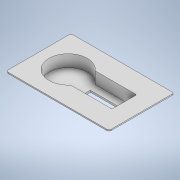
# Autodesk Inventor part: badge
Saved by Autodesk Inventor 2022 (Build 260153000, 153)
## iProperties
Created: 2019-12-22
Part Number: badge
Material: Generic
Document SubType Name: Modeling
Designer: user
Density: 1 g/cm^3
Appearance: Default
Author: user
## iProperties of the stored document _3DPrint.ipt
Created: 2019-12-23
Part Number: _3DPrint
Material: Generic
Document SubType Name: Modeling
Designer: user
Density: 1 g/cm^3
Appearance: Default
Author: user
Autodesk Inventor part; units mm, degrees
ref_plane "YZ Plane" through (0, 0, 0) normal (1, 0, 0) x (0, 1, 0)
ref_plane "XZ Plane" through (0, 0, 0) normal (0, 1, 0) x (-1, 0, 0)
ref_plane "XY Plane" through (0, 0, 0) normal (0, 0, 1) x (1, 0, 0)
sketch "Sketch1" plane through (0, 0, 0) normal (0, 1, 0) x (-1, 0, 0)
  circle A0 centre (-14.0224, -4.7987) radius 17
  line L0 (-61.8084, 4.4628) -> (-61.8084, -14.0372)
  line L1 (-59.8084, -16.0372) -> (-26.7776, -16.0372)
  line L2 (-26.7573, 6.4628) -> (-59.8084, 6.4628)
  arc A1 (-61.8084, -14.0372) -> (-59.8084, -16.0372) centre (-59.8084, -14.0372) ccw
  arc A2 (-59.8084, 6.4628) -> (-61.8084, 4.4628) centre (-59.8084, 4.4628) ccw
  line L3 (-28.2727, -0.5372) -> (-54.8084, -0.5372)
  line L4 (-54.8084, -0.5372) -> (-54.8084, -9.0372)
  line L5 (-54.8084, -9.0372) -> (-28.2727, -9.0372)
  line L6 (-28.2727, -9.0372) -> (-28.2727, -0.5372)
  line L7 (8.6213, 22.2028) -> (-72.9787, 22.2028)
  line L8 (-73.8987, -31.7772) -> (8.6213, -31.7772)
  line L9 (10.6213, -29.7772) -> (10.6213, 20.2028)
  line L10 (-74.9787, 20.2028) -> (-74.9787, 4.3773)
  line L11 (-74.9787, -30.6972) -> (-74.9787, -14.8717)
  arc A3 (-74.9787, -30.6972) -> (-73.8987, -31.7772) centre (-73.8987, -30.6972) ccw
  arc A4 (-72.9787, 22.2028) -> (-74.9787, 20.2028) centre (-72.9787, 20.2028) ccw
  arc A5 (10.6213, 20.2028) -> (8.6213, 22.2028) centre (8.6213, 20.2028) ccw
  arc A6 (8.6213, -31.7772) -> (10.6213, -29.7772) centre (8.6213, -29.7772) ccw
  line L12 (-74.9787, 4.3773) -> (-74.9787, -14.8717)
  circle A7 centre (-14.0224, -4.7987) radius 16
  line L13 (-27.4955, -15.0372) -> (-59.8084, -15.0372)
  line L14 (-60.8084, -14.0372) -> (-60.8084, 4.4628)
  arc A8 (-60.8084, -14.0372) -> (-59.8084, -15.0372) centre (-59.8084, -14.0372) ccw
  line L15 (-59.8084, 5.4628) -> (-27.576, 5.4628)
  arc A9 (-59.8084, 5.4628) -> (-60.8084, 4.4628) centre (-59.8084, 4.4628) ccw
  line L16 (-26.7776, -16.0372) -> (-25.4108, -16.0372)
  line L17 (-27.4955, -15.0372) -> (-26.3176, -15.0372)
  line L18 (-27.576, 5.4628) -> (-26.2984, 5.4628)
  line L19 (-26.7573, 6.4628) -> (-25.388, 6.4628)
  point P0 (0, 0)
  point P1 (-61.8084, -16.0372)
  dimension "d20" = 34
  dimension "d26" = 2
  dimension "d28" = 7
  dimension "d32" = 7
  dimension "d167" = 8.5
  dimension "d171" = 26.5357
  dimension "d177" = 85.6
  dimension "d229" = 32
  dimension "d230" = 1
  dimension "d231" = 1
  dimension "d232" = 1
  dimension "d233" = 1
  dimension "d234" = 1
  dimension "d235" = 1
  dimension "d241" = 53.98
  dimension "d242" = 22.74
  dimension "d243" = 22.74
  dimension "d248" = 62.786
  dimension "d249" = 6
  constraints: 40 end point, 23 point on circle, 16 tangent, 10 centre point, 6 horizontal, 6 parallel, 3 perpendicular, 3 point on line, 3 vertical, 2 equal radius
  measures "d20" diameter of A0
  measures "d26" radius of A1
  measures "d28" distance between parallel lines of L1 L5
  measures "d32" distance between parallel lines of L3 L2
  measures "d167" distance between parallel lines of L3 L5
  measures "d171" distance between parallel lines of L4 L6
  measures "d177" distance between parallel lines of L11 L9
  measures "d229" diameter of A7
  measures "d230" radial gap between concentric circles of A0 A7
  measures "d231" distance between parallel lines of L13 L1
  measures "d232" distance between parallel lines of L0 L14
  measures "d233" radius of A8
  measures "d234" distance between parallel lines of L2 L15
  measures "d235" radius of A9
  measures "d241" distance between parallel lines of L8 L7
  measures "d242" distance between parallel lines of L8 L5
  measures "d243" distance between parallel lines of L7 L3
  measures "d249" distance between parallel lines of L4 L14
extrude "Extrusion22" add sketch "Sketch1" along normal blind 1
extrude "Extrusion23" add sketch "Sketch1" against normal blind 10.5 contours A0 L16 A7 L19 | L19 A7 L18 A0 | A0 L15 A9 L14 A8 L13 L1 A1 L0 A2 L2 | A0 L13 L17 A7 L16 | L18 A7 L3 A0 | A0 L3 L4 L5 L13 A8 L14 A9 L15 | A7 L5 L6 L3 | A0 L5 A7 L17 L13 picked at (-18.1893, -4.791)
extrude "Extrusion24" cut sketch "Sketch1" against normal blind 9 contours L18 A7 L3 A0 | A0 L3 L4 L5 L13 A8 L14 A9 L15 | A7 L5 L6 L3 | A0 L5 A7 L17 L13 picked at (-18.1893, -4.791)
extrude "Extrusion25" add sketch "Sketch1" along normal blind 1 contours A0 L16 A7 L19 | L19 A7 L18 A0 | A0 L15 A9 L14 A8 L13 L1 A1 L0 A2 L2 | A0 L13 L17 A7 L16
sketch "Sketch25" plane through (0, 0, 0) normal (0, -1, 0) x (1, 0, 0)
  line L0 (61.0662, 20.9281) -> (73.8693, 20.9281) construction
  line L1 (73.8693, 20.9281) -> (73.8693, 15.5184) construction
  line L2 (73.8693, 15.5184) -> (61.0662, 15.5184) construction
  line L3 (61.0662, 15.5184) -> (61.0662, 20.9281) construction
  line L4 (63.224, 20.0701) -> (62.3275, 17.6914)
  line L5 (62.3275, 17.6914) -> (61.9679, 17.6914)
  line L6 (61.9679, 17.6914) -> (61.079, 20.0701)
  line L7 (61.079, 20.0701) -> (61.5132, 20.0701)
  line L8 (61.5132, 20.0701) -> (62.1631, 18.2385)
  line L9 (62.1631, 18.2385) -> (62.8079, 20.0701)
  line L10 (62.8079, 20.0701) -> (63.224, 20.0701)
  line L11 (65.2637, 17.6914) -> (63.7173, 17.6914)
  line L12 (63.7173, 17.6914) -> (63.7173, 18.015)
  line L13 (63.7173, 18.015) -> (64.2927, 18.015)
  line L14 (64.2927, 18.015) -> (64.2927, 20.1395)
  line L15 (64.2927, 20.1395) -> (63.7173, 20.1395)
  line L16 (63.7173, 20.1395) -> (63.7173, 20.4298)
  spline S0 degree 2 poles (63.7173, 20.4298) (64.0435, 20.4298) (64.3518, 20.6147) (64.3723, 20.8716) knots 0 0 0 1 2 2 2
  line L17 (64.3723, 20.8716) -> (64.7011, 20.8716)
  line L18 (64.7011, 20.8716) -> (64.7011, 18.015)
  line L19 (64.7011, 18.015) -> (65.2637, 18.015)
  line L20 (65.2637, 18.015) -> (65.2637, 17.6914)
  line L21 (66.5276, 17.6914) -> (66.019, 17.6914)
  line L22 (66.019, 17.6914) -> (66.019, 18.2976)
  line L23 (66.019, 18.2976) -> (66.5276, 18.2976)
  line L24 (66.5276, 18.2976) -> (66.5276, 17.6914)
  spline S1 degree 2 poles (69.1402, 19.2764) (69.1402, 18.4235) (68.6444, 17.6246) (68.128, 17.6246) knots 0 0 0 1 2 2 2
  spline S2 degree 2 poles (68.128, 17.6246) (67.604, 17.6246) (67.1133, 18.4389) (67.1133, 19.2738) knots 0 0 0 1 2 2 2
  spline S3 degree 2 poles (67.1133, 19.2738) (67.1133, 20.1318) (67.6091, 20.9256) (68.128, 20.9256) knots 0 0 0 1 2 2 2
  spline S4 degree 2 poles (68.128, 20.9256) (68.6495, 20.9256) (69.1402, 20.1035) (69.1402, 19.2764) knots 0 0 0 1 2 2 2
  spline S5 degree 2 poles (68.5956, 18.3105) (68.6572, 18.4672) (68.7086, 18.9501) (68.7086, 19.2764) knots 0 0 0 1 2 2 2
  spline S6 degree 2 poles (68.7086, 19.2764) (68.7086, 19.6026) (68.6572, 20.083) (68.593, 20.2448) knots 0 0 0 1 2 2 2
  spline S7 degree 2 poles (68.593, 20.2448) (68.5288, 20.4067) (68.3053, 20.5736) (68.128, 20.5736) knots 0 0 0 1 2 2 2
  spline S8 degree 2 poles (68.128, 20.5736) (67.9508, 20.5736) (67.7221, 20.4067) (67.6554, 20.2397) knots 0 0 0 1 2 2 2
  spline S9 degree 2 poles (67.6554, 20.2397) (67.5911, 20.0778) (67.5449, 19.5846) (67.5449, 19.2738) knots 0 0 0 1 2 2 2
  spline S10 degree 2 poles (67.5449, 19.2738) (67.5449, 18.9398) (67.586, 18.4928) (67.6528, 18.3182) knots 0 0 0 1 2 2 2
  spline S11 degree 2 poles (67.6528, 18.3182) (67.7144, 18.1538) (67.9431, 17.9765) (68.128, 17.9765) knots 0 0 0 1 2 2 2
  spline S12 degree 2 poles (68.128, 17.9765) (68.3027, 17.9765) (68.5313, 18.1435) (68.5956, 18.3105) knots 0 0 0 1 2 2 2
  line L25 (70.2268, 17.6914) -> (69.7182, 17.6914)
  line L26 (69.7182, 17.6914) -> (69.7182, 18.2976)
  line L27 (69.7182, 18.2976) -> (70.2268, 18.2976)
  line L28 (70.2268, 18.2976) -> (70.2268, 17.6914)
  line L29 (72.8214, 17.6914) -> (70.8665, 17.6914)
  line L30 (70.8665, 17.6914) -> (70.8665, 18.1409)
  spline S13 degree 2 poles (70.8665, 18.1409) (71.0771, 18.3387) (71.4522, 18.7061) (71.632, 18.9039) knots 0 0 0 1 2 2 2
  spline S14 degree 2 poles (71.632, 18.9039) (71.9942, 19.302) (72.2588, 19.7799) (72.2588, 20.0342) knots 0 0 0 1 2 2 2
  spline S15 degree 2 poles (72.2588, 20.0342) (72.2588, 20.1678) (72.1766, 20.3681) (72.1021, 20.4324) knots 0 0 0 1 2 2 2
  spline S16 degree 2 poles (72.1021, 20.4324) (72.0276, 20.4966) (71.8324, 20.5608) (71.7142, 20.5608) knots 0 0 0 1 2 2 2
  spline S17 degree 2 poles (71.7142, 20.5608) (71.6012, 20.5608) (71.37, 20.5043) (71.2646, 20.4606) knots 0 0 0 1 2 2 2
  spline S18 degree 2 poles (71.2646, 20.4606) (71.1747, 20.4246) (71.0077, 20.3219) (70.9564, 20.2859) knots 0 0 0 1 2 2 2
  line L31 (70.9564, 20.2859) -> (70.9332, 20.2859)
  line L32 (70.9332, 20.2859) -> (70.9332, 20.7381)
  spline S19 degree 2 poles (70.9332, 20.7381) (71.0643, 20.8023) (71.5344, 20.9281) (71.745, 20.9281) knots 0 0 0 1 2 2 2
  spline S20 degree 2 poles (71.745, 20.9281) (72.1894, 20.9281) (72.6904, 20.458) (72.6904, 20.0573) knots 0 0 0 1 2 2 2
  spline S21 degree 2 poles (72.6904, 20.0573) (72.6904, 19.8698) (72.603, 19.5564) (72.526, 19.4228) knots 0 0 0 1 2 2 2
  spline S22 degree 2 poles (72.526, 19.4228) (72.4489, 19.2841) (72.2254, 19.0118) (72.1021, 18.8807) knots 0 0 0 1 2 2 2
  spline S23 degree 2 poles (72.1021, 18.8807) (71.9017, 18.6624) (71.4111, 18.1949) (71.2646, 18.0587) knots 0 0 0 1 2 2 2
  line L33 (71.2646, 18.0587) -> (72.8214, 18.0587)
  line L34 (72.8214, 18.0587) -> (72.8214, 17.6914)
  point P0 (0, 0)
  constraints: 2 other
extrude "VersionNumber" cut sketch "Sketch25" against normal blind 0.5
chamfer "Chamfer1" distance 3 angle 45 6 edges at (43.2828, 0, 6.4628) (61.2226, 0, 5.877) (61.8084, 0, -4.7872) (61.2226, 0, -15.4514) (43.293, 0, -16.0372) (-2.9776, 0, -4.8141)
chamfer "Chamfer2" distance 1 angle 45 6 edges at (-2.9776, -10.5, -4.8141) (43.293, -10.5, -16.0372) (61.2226, -10.5, -15.4514) (61.8084, -10.5, -4.7872) (61.2226, -10.5, 5.877) (43.2828, -10.5, 6.4628)
body "Solid4"
